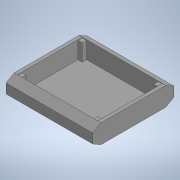
# Autodesk Inventor part: HexBody
Saved by Autodesk Inventor 2020 (Build 240168000, 168)
## iProperties
Created: 2023-12-19
Part Number: HexBody
Material: H TPU
Document SubType Name: Modeling
Designer: smz3rm
Density: 0.941117 g/cm^3
Appearance: Generic(1)
Mass: 209.726 g
Surface Area: 812.475 cm^2
Volume: 222.848 cm^3
BaseThickness: 3.000 mm
TopThickness: 1.000 mm
SideThickness: 6.000 mm
BodyWidth: 160.000 mm
BodyLength: 150.000 mm
BodyHeight: 35.000 mm
DriveMotorHeight: 17.500 mm
WheelWidth: 13.000 mm
WheelGrooveWidth: 3.000 mm
WheelGrooveDia: 25.000 mm
WheelSlotWidth: 16.500 mm
WheelDia: 50.000 mm
WheelPulleyDia: 1.000 mm
Author: smz3rm
Autodesk Inventor part; units mm, degrees
ref_plane "YZ Plane" through (0, 0, 0) normal (1, 0, 0) x (0, 1, 0)
ref_plane "XZ Plane" through (0, 0, 0) normal (0, 1, 0) x (-1, 0, 0)
ref_plane "XY Plane" through (0, 0, 0) normal (0, 0, 1) x (1, 0, 0)
sketch "Sketch1" plane through (0, 0, 0) normal (1, 0, 0) x (0, 1, 0)
  line L0 (-17.5, 75) -> (17.5, 75)
  line L1 (17.5, 75) -> (17.5, -75)
  line L2 (17.5, -75) -> (-17.5, -75)
  line L3 (-17.5, -75) -> (-17.5, 75)
  line L4 (-17.5, 75) -> (17.5, -75) construction
  line L5 (17.5, 75) -> (-17.5, -75) construction
  line L6 (-24.5, 0) -> (24.5, 0) projected
  line L7 (0, -105) -> (0, 105) projected
  line L8 (8.75, -75) -> (-8.75, -75)
  line L9 (-8.75, -75) -> (-17.5, -59.8446)
  line L10 (-17.5, -59.8446) -> (-8.75, -44.6891)
  line L11 (-8.75, -44.6891) -> (8.75, -44.6891)
  line L12 (8.75, -44.6891) -> (17.5, -59.8446)
  line L13 (17.5, -59.8446) -> (8.75, -75)
  line L14 (-8.75, 75) -> (-17.5, 59.8446)
  line L15 (17.5, 59.8446) -> (8.75, 75)
  point P0 (0, 0)
  point P1 (0, -59.8446)
  dimension "d0" = 35
  dimension "d1" = 150
  constraints: 28 end point, 4 point on line, 4 symmetric about line, 2 midpoint, 2 parallel, 1 horizontal, 1 perpendicular, 13 other
  measures "d0" distance of L1.end L2.end
  measures "d1" distance of L0.end L1.end
extrude "Extrusion1" add sketch "Sketch1" along normal mid plane 160 contours L0 L7 L6 L3 L14 | L0 L15 L1 L6 L7 | L6 L7 L11 L10 L3 | L6 L1 L12 L11 L7 | L10 L11 L7 L2 L9 | L11 L12 L13 L2 L7
sketch "Sketch2" plane through (-80, 17.5, 60.2776) normal (0, 1, 0) x (1, 0, 0)
  line L0 (160, 120.1221) -> (160, 0.433) projected
  line L1 (0, 0.433) -> (0, 120.1221) projected
  line L2 (154, 120.1221) -> (6, 120.1221)
  line L3 (6, 120.1221) -> (6, 0.433)
  line L4 (6, 0.433) -> (154, 0.433)
  line L5 (154, 0.433) -> (154, 120.1221)
  line L6 (154, 120.1221) -> (6, 0.433) construction
  line L7 (6, 120.1221) -> (154, 0.433) construction
  line L8 (0, 0.433) -> (160, 0.433) projected
  line L9 (0, 120.1221) -> (160, 120.1221) projected
  point P0 (80, 60.2776)
  dimension "d4" = 6
  constraints: 12 end point, 2 midpoint, 2 parallel, 1 horizontal, 1 perpendicular, 1 point on line
  measures "d4" distance between parallel lines of L1 L3
extrude "Extrusion2" cut sketch "Sketch2" against normal blind 32 contours L5 L4 L3 L2
sketch "Sketch3" plane through (-80, -14.5, 60.2776) normal (0, 1, 0) x (1, 0, 0)
  line L0 (6, 0.433) -> (6, 120.1221) projected
  line L1 (154, 0.433) -> (6, 0.433) projected
  line L2 (154, 120.1221) -> (154, 0.433) projected
  line L3 (6, 120.1221) -> (154, 120.1221) projected
  line L4 (6, 0.433) -> (6, 120.1221) projected
  line L5 (154, 120.1221) -> (154, 0.433) projected
  line L6 (160, 120.1221) -> (160, 0.433) projected
  line L7 (0, 0.433) -> (0, 120.1221) projected
  line L8 (6, 120.1221) -> (14, 120.1221)
  line L9 (14, 120.1221) -> (14, 112.1221)
  line L10 (14, 112.1221) -> (6, 112.1221)
  line L11 (6, 112.1221) -> (6, 120.1221)
  line L12 (-32, 60.2776) -> (192, 60.2776) projected
  line L13 (80, 165.2776) -> (80, -44.7224) projected
  line L14 (146, 120.1221) -> (146, 112.1221)
  line L15 (146, 112.1221) -> (154, 112.1221)
  line L16 (14, 0.433) -> (14, 8.433)
  line L17 (14, 8.433) -> (6, 8.433)
  line L18 (146, 0.433) -> (146, 8.433)
  line L19 (146, 8.433) -> (154, 8.433)
  line L20 (0, 120.1221) -> (6, 120.1221) projected
  line L21 (0, 0.433) -> (6, 0.433) projected
  line L22 (154, 0.433) -> (160, 0.433) projected
  line L23 (154, 120.1221) -> (160, 120.1221) projected
  point P0 (80, 60.2776)
  point P1 (14, 120.1221)
  dimension "d8" = 8
  constraints: 20 end point, 9 symmetric about line, 2 parallel, 2 perpendicular, 1 horizontal
  measures "d8" distance of L9.end L10.end
extrude "Extrusion3" add sketch "Sketch3" along normal blind 31 contours L0 L17 L16 L1 | L0 L3 L9 L10 | L18 L19 L2 L1 | L15 L14 L3 L2
equation "\"d0\" = BodyHeight"
equation "\"d1\" = BodyLength"
equation "\"d2\" = BodyWidth"
equation "\"d4\" = SideThickness"
equation "\"d5\" = BodyHeight - BaseThickness"
equation "\"d8\" = M3ScrewInsertBrim"
equation "\"d10\" = -BaseThickness + BodyHeight - TopThickness"
equation "\"BaseThickness\" = 3"
equation "\"TopThickness\" = 1"
equation "\"SideThickness\" = 6"
equation "\"BodyWidth\" = 160"
equation "\"BodyLength\" = 150"
equation "\"BodyHeight\" = 35"
equation "\"DriveMotorHeight\" = 0.5 * BodyHeight"
equation "\"WheelWidth\" = 13"
equation "\"WheelGrooveWidth\" = 3"
equation "\"WheelGrooveDia\" = 0.5 * WheelDia"
equation "\"WheelPulleyDia\" = 1"
equation "\"M3ScrewInsertBrim\" = 8"
equation "\"M3ScrewDia\" = 3.1"
equation "\"M3ScrewHeadDia\" = 6.1"
equation "\"M3ScrewInsertDia\" = 4"
equation "\"M3ScrewInsertDepth\" = 7"
equation "\"WheelDia\" = 50"
body "Solid1"
